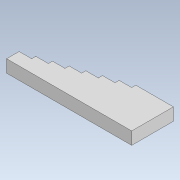
# Autodesk Inventor part: TRUC
Saved by Autodesk Inventor 2020 (Build 240168000, 168)
## iProperties
Created: 2020-07-13
Part Number: TRUC
Material: Generic
Document SubType Name: Modeling
Designer: Admin
Density: 1 g/cm^3
Appearance: Default
Author: Admin
Autodesk Inventor part; units mm, degrees
ref_plane "YZ Plane" through (0, 0, 0) normal (1, 0, 0) x (0, 1, 0)
ref_plane "XZ Plane" through (0, 0, 0) normal (0, 1, 0) x (-1, 0, 0)
ref_plane "XY Plane" through (0, 0, 0) normal (0, 0, 1) x (1, 0, 0)
sketch "Sketch1" plane through (0, 0, 0) normal (0, 1, 0) x (-1, 0, 0)
  line L0 (0, 0) -> (30, 0)
  line L1 (30, 0) -> (30, -10)
  line L2 (30, -10) -> (0, -10)
  line L3 (0, -10) -> (0, 0)
  dimension "d0" = 30
  dimension "d1" = 10
  constraints: 8 end point, 2 parallel, 1 horizontal, 1 perpendicular
  measures "d0" distance of L0.start L0.end
  measures "d1" distance of L2.end L0.start
extrude "Extrusion1" add sketch "Sketch1" along normal blind 3
sketch "Sketch2" plane through (0, 3, 0) normal (0, 1, 0) x (1, 0, 0)
  line L0 (-30, 3) -> (-27, 3)
  line L1 (-27, 3) -> (-27, 4)
  line L2 (-27, 4) -> (-24, 4)
  line L3 (-24, 4) -> (-24, 5)
  line L4 (-24, 5) -> (-21, 5)
  line L5 (-21, 5) -> (-21, 6)
  line L6 (-21, 6) -> (-18, 6)
  line L7 (-18, 6) -> (-18, 7)
  line L8 (-18, 7) -> (-15, 7)
  line L9 (-15, 7) -> (-15, 8)
  line L10 (-15, 8) -> (-12, 8)
  line L11 (-12, 8) -> (-12, 9)
  line L12 (-12, 9) -> (-9, 9)
  line L13 (-9, 9) -> (-9, 10)
  line L14 (-9, 10) -> (-1.5529, 10)
  line L15 (-1.5529, 10) -> (-1.5529, 20)
  line L16 (-1.5529, 20) -> (-30, 20)
  line L17 (-30, 20) -> (-30, 3)
  line L18 (-30, 0) -> (0, 0) projected
  line L19 (-30, 10) -> (-30, 0) projected
  dimension "d4" = 3
  dimension "d5" = 3
  dimension "d6" = 3
  dimension "d7" = 3
  dimension "d8" = 3
  dimension "d9" = 3
  dimension "d10" = 1
  dimension "d11" = 1
  dimension "d12" = 1
  dimension "d13" = 1
  dimension "d14" = 1
  dimension "d15" = 1
  dimension "d16" = 3
  dimension "d17" = 1
  dimension "d18" = 3
  dimension "d19" = 10
  dimension "d20" = 28.4471
  constraints: 36 end point, 16 perpendicular, 1 horizontal, 1 point on line, 1 vertical
  measures "d4" distance of L0.start L0.end
  measures "d5" distance of L1.end L2.end
  measures "d6" distance of L3.end L4.end
  measures "d7" distance of L5.end L6.end
  measures "d8" distance of L7.end L8.end
  measures "d9" distance of L9.end L10.end
  measures "d10" distance of L0.end L1.end
  measures "d11" distance of L2.end L3.end
  measures "d12" distance of L4.end L5.end
  measures "d13" distance of L6.end L7.end
  measures "d14" distance of L8.end L9.end
  measures "d15" distance of L10.end L11.end
  measures "d16" distance of L11.end L12.end
  measures "d17" distance of L12.end L13.end
  measures "d18" distance between parallel lines of L0 L18
  measures "d19" distance of L14.end L15.end
  measures "d20" distance of L15.end L16.end
extrude "Extrusion2" cut sketch "Sketch2" against normal through all
body "Solid1"
